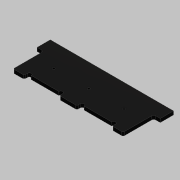
# Autodesk Inventor part: AK-C-C39-Pinhole-Board
Saved by Autodesk Inventor 2016 (Build 200138000, 138)
## iProperties
Created: 2016-05-19
Part Number: AK-C-C39-Pinhole-Board
Material: Generic
Document SubType Name: Modeling
Designer: admin
Density: 1 g/cm^3
Appearance: Glossy - Black
Author: admin
Autodesk Inventor part; units mm, degrees
ref_plane "YZ Plane" through (0, 0, 0) normal (1, 0, 0) x (0, 1, 0)
ref_plane "XZ Plane" through (0, 0, 0) normal (0, 1, 0) x (-1, 0, 0)
ref_plane "XY Plane" through (0, 0, 0) normal (0, 0, 1) x (1, 0, 0)
sketch "Sketch1" plane through (0, 0, 0) normal (0, 0, 1) x (1, 0, 0)
  line L0 (-28, 9.2) -> (28, 9.2)
  line L1 (28, 9.2) -> (28, 3.2)
  line L2 (28, 3.2) -> (25.875, 3.2)
  line L3 (25, 2.325) -> (25, -10.2)
  line L4 (24.5, -10.7) -> (20.5, -10.7)
  line L5 (20, -10.2) -> (20, -9.2)
  line L6 (18.25, -9.2) -> (5.75, -9.2)
  line L7 (4, -9.2) -> (4, -10.2)
  line L8 (3.5, -10.7) -> (-3.5, -10.7)
  line L9 (-4, -10.2) -> (-4, -9.2)
  line L10 (-5.75, -9.2) -> (-18.25, -9.2)
  line L11 (-20, -9.2) -> (-20, -10.2)
  line L12 (-20.5, -10.7) -> (-24.5, -10.7)
  line L13 (-25, -10.2) -> (-25, 2.325)
  line L14 (-25.875, 3.2) -> (-28, 3.2)
  line L15 (-28, 3.2) -> (-28, 9.2)
  line L16 (0, 7.251) -> (0, -4.9434) construction
  line L17 (-9.4671, 0) -> (8.147, 0) construction
  arc A0 (-18.25, -9.2) -> (-20, -9.2) centre (-19.125, -9.2) ccw
  arc A1 (-4, -9.2) -> (-5.75, -9.2) centre (-4.875, -9.2) ccw
  arc A2 (5.75, -9.2) -> (4, -9.2) centre (4.875, -9.2) ccw
  arc A3 (20, -9.2) -> (18.25, -9.2) centre (19.125, -9.2) ccw
  arc A4 (-25, 2.325) -> (-25.875, 3.2) centre (-25.875, 2.325) ccw
  arc A5 (25.875, 3.2) -> (25, 2.325) centre (25.875, 2.325) ccw
  line L18 (-25, -10.2) -> (-24.5, -10.7)
  line L19 (-20, -10.2) -> (-20.5, -10.7)
  line L20 (-4, -10.2) -> (-3.5, -10.7)
  line L21 (3.5, -10.7) -> (4, -10.2)
  line L22 (20, -10.2) -> (20.5, -10.7)
  line L23 (25, -10.2) -> (24.5, -10.7)
  point P0 (0, 0)
  dimension "d0" = 8
  dimension "d1" = 1.5
  dimension "d2" = 5
  dimension "d3" = 20
  dimension "d4" = 18.4
  dimension "d5" = 1.75
  dimension "d6" = 6
  dimension "d7" = 3
  dimension "d19" = 45
  dimension "d20" = 0.5
  constraints: 48 end point, 12 point on circle, 9 vertical, 8 point on line, 8 tangent, 7 horizontal, 6 centre point, 6 equal length, 5 equal radius, 4 parallel, 3 collinear, 1 perpendicular, 4 other
  measures "d0" distance between parallel lines of L7 L9
  measures "d1" distance between parallel lines of L8 L10
  measures "d2" distance between parallel lines of L11 L13
  measures "d3" distance between parallel lines of L11 L16
  measures "d4" distance between parallel lines of L6 L0
  measures "d5" diameter of A0
  measures "d6" distance between parallel lines of L2 L0
  measures "d7" distance between parallel lines of L13 L15
  measures "d19" angle of L12 L18
  measures "d20" distance from line of L12.end L13
extrude "Extrusion1" add sketch "Sketch1" along normal blind 1.6
sketch "Sketch2" plane through (0, 0, 1.6) normal (0, 0, 1) x (1, 0, 0)
  line L0 (-28, 9.2) -> (28, 9.2) projected
  point P0 (0, 0)
  point P1 (0, -1.3)
  point P2 (-16, -1.3)
  point P3 (16, -1.3)
  dimension "d10" = 16
  dimension "d11" = 16
  dimension "d21" = 10.5
  constraints: 2 horizontal alignment, 1 vertical alignment
  measures "d10" distance of point (0, -1.3) point (-16, -1.3)
  measures "d11" distance of point (16, -1.3) point (0, -1.3)
  measures "d21" distance from line of point (-16, -1.3) L0
hole "Hole1" at (0, -1.3, 1.6) at (-16, -1.3, 1.6) at (16, -1.3, 1.6) direction (0, 0, -1) diameter 1 end through all
body "Solid1"
